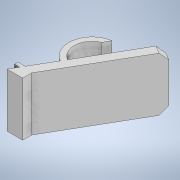
# Autodesk Inventor part: part_v3-4_3
Saved by Autodesk Inventor 2021 (Build 250183000, 183)
## iProperties
Created: 2023-04-16
Part Number: part_v3-4_3
Material: Generic
Document SubType Name: Modeling
Designer: malo
Density: 1 g/cm^3
Appearance: Default
Author: malo
Autodesk Inventor part; units mm, degrees
ref_plane "YZ Plane" through (0, 0, 0) normal (1, 0, 0) x (0, 1, 0)
ref_plane "XZ Plane" through (0, 0, 0) normal (0, 1, 0) x (-1, 0, 0)
ref_plane "XY Plane" through (0, 0, 0) normal (0, 0, 1) x (1, 0, 0)
sketch "Sketch22" plane through (0, 0, 0) normal (0, 1, 0) x (-1, 0, 0)
  line L0 (0, 0) -> (-4.3301, 0)
  line L1 (-4.3301, 0) -> (-4.3301, -2.5)
  line L2 (-4.3301, -2.5) -> (-18.3309, -26.75)
  line L3 (-18.3309, -26.75) -> (-16.1658, -28)
  line L4 (-16.1658, -28) -> (0, 0)
  dimension "d180" = 60
  dimension "d182" = 2.5
  dimension "d184" = 2.5
  dimension "d185" = 28
  constraints: 10 end point, 3 perpendicular, 1 horizontal
  measures "d180" angle of L0 L4
  measures "d182" distance of L0.end L1.end
  measures "d184" distance between parallel lines of L4 L2
  measures "d185" vertical distance of L3.end L0.start
extrude "Extrusion22" add sketch "Sketch22" along normal blind 15
sketch "Sketch23" plane through (0, 15, 0) normal (0, 1, 0) x (1, 0, 0)
  line L0 (16.1658, 28) -> (0, 0) projected
  arc A0 (6.7017, 19.6077) -> (6.1658, 10.6795) centre (8.6658, 15.0096) ccw
  arc A1 (7.7634, 21.4467) -> (5.4158, 9.3805) centre (8.6658, 15.0096) ccw
  line L1 (18.3309, 26.75) -> (16.1658, 28) projected
  line L2 (6.7017, 19.6077) -> (7.7634, 21.4467)
  dimension "d188" = 10
  dimension "d189" = 1.5
  dimension "d190" = 15
  dimension "d191" = 4
  constraints: 4 point on circle, 3 point on line, 2 centre point, 2 end point, 1 coincident, 1 parallel
  measures "d188" diameter of A0
  measures "d189" radial gap between concentric circles of A1 A0
  measures "d190" distance from line of A0.centre L1
  measures "d191" distance between parallel lines of L0 L2
extrude "Extrusion23" add sketch "Sketch23" against normal blind 15
sketch "Sketch24" plane through (0, 15, 0) normal (0, 1, 0) x (1, 0, 0)
  line L0 (4.3301, 0) -> (4.3301, 2.5) projected
  line L1 (4.3301, 2.2) -> (-0.1525, 2.2)
  line L2 (0, 0) -> (4.3301, 0) projected
  line L3 (-0.1525, 2.2) -> (-0.1525, 3.2)
  line L4 (-0.1525, 3.2) -> (1.8475, 3.2)
  line L5 (1.8475, 3.2) -> (1.2702, 2.2)
  line L6 (5.4158, 9.3805) -> (0, 0) projected
  dimension "d194" = 2.2
  dimension "d195" = 2
  dimension "d196" = 1
  constraints: 8 end point, 4 point on line, 1 horizontal, 1 perpendicular, 1 vertical
  measures "d194" distance between parallel lines of L2 L1
  measures "d195" distance of L3.end L4.end
  measures "d196" distance of L1.end L3.end
extrude "Extrusion24" add sketch "Sketch24" against normal blind 4 contours L1 L3 L4 L5
chamfer "Chamfer6" distance 2 angle 45 2 edges at (17.2483, 15, -27.375) (17.2483, 0, -27.375)
body "Solid1"
